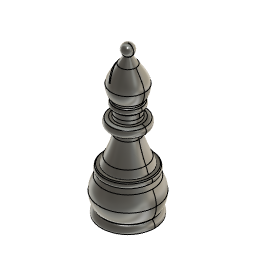
Bishop v2 (Autodesk Fusion 360 design; units mm, degrees)
Autodesk Fusion 360 part; units mm, degrees
sketch "side view" plane through (0, 0, 0) normal (0, 1, 0) x (1, 0, 0)
  spline S0 degree 3 poles (23.6538, -103.9328) (22.6219, -103.483) (21.7488, -102.3718) (21.5371, -101.2605) knots 0 0 0 0 1 1 1 1
  spline S1 degree 3 poles (21.5371, -101.2605) (21.3783, -100.308) (22.225, -97.9532) (22.7277, -97.9532) knots 0 0 0 0 1 1 1 1
  spline S2 degree 3 poles (22.7277, -97.9532) (23.3892, -97.9532) (22.9129, -96.6303) (21.5635, -94.7782) knots 0 0 0 0 1 1 1 1
  spline S3 degree 3 poles (21.5635, -94.7782) (20.5317, -93.376) (20.1083, -92.5557) (20.1083, -91.9737) knots 0 0 0 0 1 1 1 1
  spline S4 degree 3 poles (20.1083, -91.9737) (20.1083, -91.5239) (20.6375, -90.0157) (21.2725, -88.6399) knots 0 0 0 0 1 1 1 1
  spline S5 degree 3 poles (21.2725, -88.6399) (22.7542, -85.4649) (22.9658, -84.7241) (22.3573, -84.7241) knots 0 0 0 0 1 1 1 1
  spline S6 degree 3 poles (22.3573, -84.7241) (22.0663, -84.7241) (21.5635, -85.5178) (20.7698, -87.1847) knots 0 0 0 0 1 1 1 1
  spline S7 degree 3 poles (20.7698, -87.1847) (20.1348, -88.5076) (19.4469, -89.8305) (19.2617, -90.1216) knots 0 0 0 0 1 1 1 1
  spline S8 degree 3 poles (19.2617, -90.1216) (18.8913, -90.5714) (18.8383, -90.5449) (18.0975, -89.5924) knots 0 0 0 0 1 1 1 1
  spline S9 degree 3 poles (18.0975, -89.5924) (16.9069, -88.0314) (15.1871, -85.0151) (14.7108, -83.5864) knots 0 0 0 0 1 1 1 1
  spline S10 degree 3 poles (14.7108, -83.5864) (13.8906, -81.1522) (14.3404, -78.3741) (16.166, -74.7757) knots 0 0 0 0 1 1 1 1
  line L0 (16.166, -74.7757) -> (17.2508, -72.6326)
  line L1 (17.2508, -72.6326) -> (16.6952, -71.5478)
  spline S11 degree 3 poles (16.6952, -71.5478) (15.9808, -70.1455) (16.0073, -69.8016) (16.8275, -69.1401) knots 0 0 0 0 1 1 1 1
  spline S12 degree 3 poles (16.8275, -69.1401) (17.5154, -68.611) (17.8329, -68.5845) (25.2677, -68.5845) knots 0 0 0 0 1 1 1 1
  line L2 (25.2677, -68.5845) -> (32.9935, -68.5845)
  line L3 (32.9935, -68.5845) -> (33.6021, -69.2195)
  spline S13 degree 3 poles (33.6021, -69.2195) (34.3694, -70.0662) (34.3694, -71.0716) (33.5756, -71.9182) knots 0 0 0 0 1 1 1 1
  line L4 (33.5756, -71.9182) -> (32.9406, -72.5797)
  line L5 (32.9406, -72.5797) -> (33.9196, -74.3524)
  spline S14 degree 3 poles (33.9196, -74.3524) (35.3219, -76.9453) (35.7981, -78.8503) (35.6658, -81.3374) knots 0 0 0 0 1 1 1 1
  spline S15 degree 3 poles (35.6658, -81.3374) (35.5071, -84.0362) (34.4223, -86.2322) (30.1096, -92.688) knots 0 0 0 0 1 1 1 1
  line L6 (30.1096, -92.688) -> (26.9081, -97.4505)
  line L7 (26.9081, -97.4505) -> (27.6225, -98.1914)
  spline S16 degree 3 poles (27.6225, -98.1914) (30.4006, -101.0753) (27.3315, -105.5203) (23.6538, -103.9328) knots 0 0 0 0 1 1 1 1
  spline S17 degree 3 poles (18.071, -67.7378) (17.9652, -67.5526) (17.8065, -66.2562) (17.7271, -64.8803) knots 0 0 0 0 1 1 1 1
  line L8 (17.7271, -64.8803) -> (17.5948, -62.3668)
  line L9 (17.5948, -62.3668) -> (16.5365, -62.2874)
  spline S18 degree 3 poles (16.5365, -62.2874) (14.7373, -62.1816) (14.2875, -61.9964) (13.7583, -61.0968) knots 0 0 0 0 1 1 1 1
  spline S19 degree 3 poles (13.7583, -61.0968) (12.7265, -59.4035) (13.2556, -57.4985) (14.9754, -56.7841) knots 0 0 0 0 1 1 1 1
  spline S20 degree 3 poles (14.9754, -56.7841) (16.2983, -56.2285) (33.999, -56.2549) (35.3219, -56.7841) knots 0 0 0 0 1 1 1 1
  spline S21 degree 3 poles (35.3219, -56.7841) (37.121, -57.5514) (37.5444, -60.0914) (36.0892, -61.4672) knots 0 0 0 0 1 1 1 1
  spline S22 degree 3 poles (36.0892, -61.4672) (35.5865, -61.917) (35.0044, -62.1287) (33.9196, -62.2345) knots 0 0 0 0 1 1 1 1
  line L10 (33.9196, -62.2345) -> (32.4115, -62.3668)
  line L11 (32.4115, -62.3668) -> (32.385, -64.6157)
  spline S23 degree 3 poles (32.385, -64.6157) (32.385, -65.8593) (32.3585, -67.1293) (32.3321, -67.4732) knots 0 0 0 0 1 1 1 1
  line L12 (32.3321, -67.4732) -> (32.2792, -68.0553)
  line L13 (32.2792, -68.0553) -> (25.2942, -68.0553)
  spline S24 degree 3 poles (25.2942, -68.0553) (19.976, -68.0553) (18.2298, -67.976) (18.071, -67.7378) knots 0 0 0 0 1 1 1 1
  spline S25 degree 3 poles (18.9177, -55.6464) (18.8383, -55.4876) (18.6531, -54.4028) (18.4944, -53.1857) knots 0 0 0 0 1 1 1 1
  spline S26 degree 3 poles (18.4944, -53.1857) (18.1769, -50.5664) (16.1396, -44.2693) (14.261, -40.0095) knots 0 0 0 0 1 1 1 1
  spline S27 degree 3 poles (14.261, -40.0095) (13.5202, -38.3426) (12.6735, -36.3847) (12.356, -35.6968) knots 0 0 0 0 1 1 1 1
  spline S28 degree 3 poles (12.356, -35.6968) (11.8798, -34.612) (11.8533, -34.4003) (12.1708, -34.1887) knots 0 0 0 0 1 1 1 1
  spline S29 degree 3 poles (12.1708, -34.1887) (12.409, -34.0299) (17.8065, -33.9241) (25.0296, -33.9241) knots 0 0 0 0 1 1 1 1
  spline S30 degree 3 poles (25.0296, -33.9241) (35.1367, -33.9241) (37.5708, -34.0035) (37.9677, -34.2945) knots 0 0 0 0 1 1 1 1
  spline S31 degree 3 poles (37.9677, -34.2945) (38.444, -34.6385) (38.3646, -34.8501) (36.5919, -38.8453) knots 0 0 0 0 1 1 1 1
  spline S32 degree 3 poles (36.5919, -38.8453) (34.2635, -44.0312) (32.7025, -48.5555) (32.1469, -51.5982) knots 0 0 0 0 1 1 1 1
  spline S33 degree 3 poles (32.1469, -51.5982) (31.9088, -52.8682) (31.5913, -54.3499) (31.459, -54.9055) knots 0 0 0 0 1 1 1 1
  line L14 (31.459, -54.9055) -> (31.1944, -55.8845)
  line L15 (31.1944, -55.8845) -> (25.1354, -55.8845)
  spline S34 degree 3 poles (25.1354, -55.8845) (21.6694, -55.8845) (19.0235, -55.7787) (18.9177, -55.6464) knots 0 0 0 0 1 1 1 1
  spline S35 degree 3 poles (10.0013, -33.3949) (9.2604, -32.9451) (8.89, -31.437) (9.3133, -30.5639) knots 0 0 0 0 1 1 1 1
  line L16 (9.3133, -30.5639) -> (9.6573, -29.823)
  line L17 (9.6573, -29.823) -> (24.8179, -29.7437)
  spline S36 degree 3 poles (24.8179, -29.7437) (39.661, -29.6907) (39.9521, -29.6907) (40.4813, -30.2199) knots 0 0 0 0 1 1 1 1
  spline S37 degree 3 poles (40.4813, -30.2199) (41.1427, -30.8814) (41.1692, -32.0985) (40.5077, -32.8922) knots 0 0 0 0 1 1 1 1
  line L18 (40.5077, -32.8922) -> (40.005, -33.5272)
  line L19 (40.005, -33.5272) -> (25.2148, -33.5801)
  spline S38 degree 3 poles (25.2148, -33.5801) (15.8221, -33.633) (10.2923, -33.5537) (10.0013, -33.3949) knots 0 0 0 0 1 1 1 1
  spline S39 degree 3 poles (10.1865, -28.3414) (9.1017, -27.3624) (7.0644, -23.4201) (6.4823, -21.0918) knots 0 0 0 0 1 1 1 1
  spline S40 degree 3 poles (6.4823, -21.0918) (5.6885, -17.9697) (6.2177, -13.2337) (7.6465, -10.4026) knots 0 0 0 0 1 1 1 1
  spline S41 degree 3 poles (7.6465, -10.4026) (8.6783, -8.4182) (7.62, -8.5241) (24.5269, -8.5241) knots 0 0 0 0 1 1 1 1
  spline S42 degree 3 poles (24.5269, -8.5241) (33.7079, -8.5241) (39.9256, -8.6299) (40.3225, -8.7887) knots 0 0 0 0 1 1 1 1
  spline S43 degree 3 poles (40.3225, -8.7887) (41.8835, -9.3707) (43.4446, -13.657) (43.471, -17.3876) knots 0 0 0 0 1 1 1 1
  spline S44 degree 3 poles (43.471, -17.3876) (43.471, -20.3774) (43.0213, -22.0443) (41.0633, -26.0395) knots 0 0 0 0 1 1 1 1
  line L20 (41.0633, -26.0395) -> (39.5552, -29.1351)
  line L21 (39.5552, -29.1351) -> (25.3471, -29.1351)
  line L22 (25.3471, -29.1351) -> (11.139, -29.1616)
  line L23 (11.139, -29.1616) -> (10.1865, -28.3414)
  spline S45 degree 3 poles (8.7313, -7.9155) (7.6465, -7.5451) (6.8792, -6.2487) (6.8792, -4.767) knots 0 0 0 0 1 1 1 1
  spline S46 degree 3 poles (6.8792, -4.767) (6.8792, -4.0526) (7.0379, -3.7087) (7.3819, -3.497) knots 0 0 0 0 1 1 1 1
  spline S47 degree 3 poles (7.3819, -3.497) (8.1756, -3.1001) (41.8571, -3.1266) (42.2804, -3.5499) knots 0 0 0 0 1 1 1 1
  spline S48 degree 3 poles (42.2804, -3.5499) (43.18, -4.4495) (42.201, -7.1747) (40.7458, -7.9155) knots 0 0 0 0 1 1 1 1
  spline S49 degree 3 poles (40.7458, -7.9155) (39.8463, -8.3918) (10.1071, -8.3653) (8.7313, -7.9155) knots 0 0 0 0 1 1 1 1
  line L24 (24.9171, -3.2158) -> (24.9171, -104.2549)
  constraint coincident S47 L24.start
  constraint coincident S16 L24.end
  constraint vertical L24
revolve "Revolve1" add sketch "side view" angle 360 about axis through (24.9171, 0, 3.2158) along (0, 0, 1) contours S12 L2 L3 S13 L4 L5 S14 S15 L6 L7 S16 L24 | S20 S21 S22 L10 L11 S23 L12 L13 S24 L24 | S29 S30 S31 S32 S33 L14 L15 S34 L24 | S36 S37 L18 L19 S38 L24 | S42 S43 S44 L20 L21 L22 L24 | S47 S48 S49 L24 makes body 1 at (16.7526, 7.3883, 29.7297) makes body 2 at (34.1161, -1.8596, 85.8905) makes body 3 at (43.1339, -2.7457, 15.5157) makes body 4 at (34.4208, -1.4324, 43.7803) makes body 5 at (15.0804, 6.8877, 58.8952) makes body 6 at (18.244, -4.0209, 3.2548)
sketch "top cut" plane through (0, 0, 0) normal (0, 1, 0) x (1, 0, 0)
  line L0 (18, -92) -> (22, -85)
  line L1 (22, -85) -> (22.3018, -84.7324)
  line L2 (22.3018, -84.7324) -> (22.6, -84.8)
  line L3 (22.6, -84.8) -> (22.6726, -85.0479)
  line L4 (22.6726, -85.0479) -> (22.6363, -85.296)
  line L5 (22.6363, -85.296) -> (19.3937, -93.2694)
  line L6 (19.3937, -93.2694) -> (18, -92)
extrude "Extrude1" cut sketch "top cut" along normal blind 20 and the other way blind 25 bodies 2
move_body "Align1" bodies 3 to x (1, 0, 0) y (0, 1, 0) z (0, 0, 1) at (0, 0, -0.8731)
move_body "Align2" bodies 1 to x (1, 0, 0) y (0, 1, 0) z (0, 0, 1) at (0, 0, -1.9579)
move_body "Align3" bodies 4 to x (1, 0, 0) y (0, 1, 0) z (0, 0, 1) at (0, 0, -2.7252)
move_body "Align4" bodies 5 to x (1, 0, 0) y (0, 1, 0) z (0, 0, 1) at (0, 0, -3.6248)
move_body "Align5" bodies 2 to x (1, 0, 0) y (0, 1, 0) z (0, 0, 1) at (0, 0, -4.154)
combine "Combine1" operation add target body 1 tool bodies 2 3 4 5 6
named bodies: "bishop"
